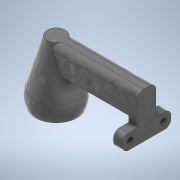
# Autodesk Inventor part: BallFemale
Saved by Autodesk Inventor 2022 (Build 260153000, 153)
## iProperties
Created: 2021-11-09
Part Number: BallFemale
Material: Generic
Document SubType Name: Modeling
Designer: Juan
Density: 1 g/cm^3
Appearance: Default
Author: Juan
Autodesk Inventor part; units mm, degrees
ref_plane "XZ Plane" through (0, 0, 0) normal (0, 1, 0) x (-1, 0, 0)
ref_plane "XY Plane" through (0, 0, 0) normal (0, 0, 1) x (1, 0, 0)
sketch "Sketch1" plane through (0, 0, 0) normal (1, 0, 0) x (0, 1, 0)
  arc A0 (7.4985, -0.1486) -> (-3.2805, 6.7445) centre (0, 0) ccw
  line L0 (0, 0) -> (-1.75, 0)
  line L1 (-1.75, 0) -> (-1.75, -0.1486)
  line L2 (-1.75, -4.1458) -> (-0.74, -4.1458) construction
  line L3 (-3.2805, 6.7445) -> (-3.0298, 6.3103)
  line L4 (-3.2805, 6.7445) -> (-2.7791, 6.7445) construction
  line L5 (6.9984, -0.1486) -> (16.9984, -0.1486)
  line L6 (16.9984, -0.1486) -> (16.9984, 2.8514)
  line L7 (16.9984, 2.8514) -> (1.2284, 7.4544)
  arc A1 (6.9984, -0.1486) -> (-3.0298, 6.3103) centre (0, 0) ccw
  point P0 (2.1014, 7.1996)
  dimension "d1" = 15
  dimension "d2" = 1.75
  dimension "d4" = 60
  dimension "d5" = 10
  dimension "d6" = 3
  dimension "d8" = 7
  constraints: 16 end point, 4 horizontal, 4 point on circle, 3 point on line, 2 centre point, 2 coincident, 1 equal length, 1 perpendicular, 1 tangent, 1 vertical
  measures "d1" diameter of A0
  measures "d2" distance of L0.start L0.end
  measures "d4" angle of L3 L4
  measures "d5" distance of L5.start L5.end
  measures "d6" distance of L5.end L6.end
  measures "d8" radius of A1
revolve "Revolution1" add sketch "Sketch1" angle 360 about axis through (0, 6.9984, -0.1486) along (0, 1, 0)
ref_plane "Work Plane1" through (30, 0, 0) normal (1, 0, 0) x (0, 1, 0)
sketch "Sketch2" plane through (30, 0, 0) normal (1, 0, 0) x (0, 1, 0)
  line L0 (16.9984, -3.1486) -> (16.9984, 2.8514) projected
  line L1 (14.9984, 2.8514) -> (6.9984, 2.8514)
  line L2 (14.9984, -3.1486) -> (6.9984, -3.1486)
  line L3 (16.9984, 0.8514) -> (16.9984, -1.1486)
  arc A0 (16.9984, 0.8514) -> (14.9984, 2.8514) centre (14.9984, 0.8514) ccw
  arc A1 (14.9984, -3.1486) -> (16.9984, -1.1486) centre (14.9984, -1.1486) ccw
  line L4 (6.9984, 2.8514) -> (6.9984, 7.8514)
  line L5 (6.9984, 7.8514) -> (1.9984, 7.8514)
  line L6 (1.9984, 7.8514) -> (1.9984, -8.1486)
  line L7 (2.1014, -7.4967) -> (2.1014, 7.1996) projected
  line L8 (1.9984, 7.8514) -> (17.9984, 7.8514) construction
  line L9 (1.9984, -8.1486) -> (6.9984, -8.1486)
  line L10 (6.9984, -8.1486) -> (6.9984, -3.1486)
  point P0 (0, 0)
  dimension "d10" = 10
  dimension "d11" = 10
  dimension "d12" = 2
  dimension "d13" = 5
  dimension "d14" = 5
  dimension "d15" = 16
  dimension "d16" = 90
  dimension "d17" = 5
  constraints: 18 end point, 4 point on circle, 4 point on line, 4 tangent, 3 horizontal, 2 centre point, 2 parallel, 2 perpendicular, 2 vertical, 1 equal radius
  measures "d10" distance of L0.end L1.end
  measures "d11" distance of L0.start L2.end
  measures "d12" radius of A0
  measures "d13" distance of L1.end L4.end
  measures "d14" distance of L4.end L5.end
  measures "d15" distance of L5.end L6.end
  measures "d16" angle of L6 L8
  measures "d17" distance of L6.end L9.end
extrude "Extrusion1" add sketch "Sketch2" against normal blind 3
sketch "Sketch3" plane through (27, 0, 0) normal (-1, 0, 0) x (0, 0, 1)
  line L0 (0.8514, 16.9984) -> (-1.1486, 16.9984) projected
  line L1 (-0.1486, 16.9984) -> (-0.1486, 8.9984)
  line L2 (-0.1486, 8.9984) -> (-3.1486, 8.9984)
  line L3 (-3.1486, 14.9984) -> (-3.1486, 6.9984) projected
  line L4 (-0.1486, 8.9984) -> (2.8514, 8.9984)
  line L5 (2.8514, 6.9984) -> (2.8514, 14.9984) projected
  arc A0 (2.8514, 14.9984) -> (0.8514, 16.9984) centre (0.8514, 14.9984) ccw projected
  arc A1 (-1.1486, 16.9984) -> (-3.1486, 14.9984) centre (-1.1486, 14.9984) ccw projected
  point P0 (0, 0)
  dimension "d20" = 8
  constraints: 6 end point, 3 point on line, 1 midpoint, 1 perpendicular, 1 vertical
  measures "d20" distance of L1.start L1.end
extrude "Extrusion2" add sketch "Sketch3" along normal up to surface
fillet "Fillet1" radius 2 4 edges at (28.5, 1.9984, -8.1486) (28.5, 6.9984, -8.1486) (28.5, 1.9984, 7.8514) (28.5, 6.9984, 7.8514)
sketch "Sketch4" plane through (30, 0, 0) normal (1, 0, 0) x (0, 0, -1)
  line L0 (8.1486, 4.9984) -> (8.1486, 3.9984) projected
  line L1 (8.1486, 4.4984) -> (5.6486, 4.4984)
  circle A0 centre (5.6486, 4.4984) radius 1
  line L2 (-7.8514, 4.9984) -> (-7.8514, 3.9984) projected
  line L3 (-7.8514, 4.4984) -> (-5.3514, 4.4984)
  circle A1 centre (-5.3514, 4.4984) radius 1
  point P0 (0, 0)
  dimension "d24" = 2.5
  dimension "d25" = 2
  dimension "d26" = 2.5
  dimension "d27" = 2
  constraints: 4 end point, 2 centre point, 2 coincident, 2 horizontal, 2 midpoint
  measures "d24" distance of L1.start L1.end
  measures "d25" diameter of A0
  measures "d26" distance of L3.start L3.end
  measures "d27" diameter of A1
extrude "Extrusion3" cut sketch "Sketch4" against normal up to surface (3 mm away)
sketch "Sketch5" plane through (27, 0, 0) normal (-1, 0, 0) x (0, 0, 1)
  circle A0 centre (5.3514, 4.4984) radius 1 projected
  circle A1 centre (-5.6486, 4.4984) radius 1 projected
  circle A2 centre (-5.6486, 4.4984) radius 1.7
  circle A3 centre (5.3514, 4.4984) radius 1.7
  point P0 (0, 0)
  dimension "d30" = 3.4
  dimension "d31" = 3.4
  constraints: 2 centre point, 2 coincident
  measures "d30" diameter of A2
  measures "d31" diameter of A3
extrude "Extrusion4" cut sketch "Sketch5" against normal blind 1.5
equation "\"d21\" = d20"
body "Solid1"
